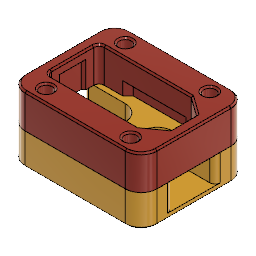
Wiring Box v13 (Autodesk Fusion 360 archive; units mm, degrees)
design "XT90 Mount"
Autodesk Fusion 360 part; units mm, degrees
sketch "Sketch1" plane through (0, 0, 0) normal (0, 0, 1) x (1, 0, 0) in component "Top"
  line L0 (12.5, -10) -> (-12.5, -10)
  line L1 (-12.5, -10) -> (-12.5, 10)
  line L2 (-12.5, 10) -> (12.5, 10)
  line L3 (12.5, 10) -> (12.5, -10)
  line L4 (12.5, -10) -> (-12.5, 10) construction
  line L5 (-12.5, -10) -> (12.5, 10) construction
  line L6 (-10.5, 5) -> (-10.5, -5)
  line L7 (-10.5, -5) -> (7, -5)
  line L8 (7, -5) -> (10.5, -2.5)
  line L9 (10.5, -2.5) -> (10.5, 2.5)
  line L10 (10.5, 2.5) -> (7, 5)
  line L11 (7, 5) -> (-10.5, 5)
  line L12 (0, 0) -> (-22, 0) construction
  line L13 (0, 0) -> (0, 9) construction
  dimension "d1" = 25
  dimension "d2" = 20
  dimension "d3" = 10
  dimension "d4" = 21
  dimension "d5" = 2.5
  dimension "d6" = 3.5
  constraint horizontal L0
  constraint perpendicular L0 L1
  constraint parallel L0 L2
  constraint parallel L1 L3
  constraint coincident L4 L12.start
  constraint coincident L5 L12.start
  constraint coincident L12.start L13.start
  constraint vertical L6
  constraint horizontal L11
  constraint horizontal L7
  constraint vertical L9
  constraint horizontal L12
  constraint symmetric L7 L11 L12
  constraint perpendicular L12 L13
  constraint symmetric L8 L10 L12
  measures "d1" distance of L1.end L2.end
  measures "d2" distance of L0.end L1.end
  measures "d3" distance of L6.start L6.end
  measures "d4" distance of L6 L9
  measures "d5" vertical distance of L9.end L10.end
  measures "d6" horizontal distance of L9.end L10.end
extrude "Extrude1" add sketch "Sketch1" against normal blind 1.5 makes body 1 in component "Top"
fillet "Fillet1" radius 1 2 edges at (-10.5, 5, -0.75) (-10.5, -5, -0.75) on bodies 1 in component "Top"
sketch "Sketch2" plane through (0, 0, -1.5) normal (0, 0, -1) x (1, 0, 0) in component "Top"
  line L0 (7, -5) -> (-9.5, -5)
  arc A0 (-10.5, -4) -> (-9.5, -5) centre (-9.5, -4) ccw
  line L1 (-10.5, -4) -> (-10.5, 4)
  arc A1 (-9.5, 5) -> (-10.5, 4) centre (-9.5, 4) ccw
  line L2 (-9.5, 5) -> (7, 5)
  line L3 (7, 5) -> (10.5, 2.5)
  line L4 (10.5, 2.5) -> (10.5, -2.5)
  line L5 (10.5, -2.5) -> (7, -5)
  line L6 (-12.5, -10) -> (12.5, -10)
  line L7 (12.5, -10) -> (12.5, 10)
  line L8 (12.5, 10) -> (-12.5, 10)
  line L9 (-12.5, 10) -> (-12.5, -10)
  line L10 (10.5, 2.5) -> (11, 2.1429)
  line L11 (11, 2.1429) -> (11, -2.1429)
  line L12 (11, -2.1429) -> (10.5, -2.5)
  line L13 (0, 0) -> (0, 13.3423) construction
  line L14 (-10.5, 2.5) -> (-11, 2.1429)
  line L15 (-11, 2.1429) -> (-11, -2.1429)
  line L16 (-11, -2.1429) -> (-10.5, -2.5)
  dimension "d11" = 0.5
  constraint coincident L3.end L4.start
  constraint parallel L3 L10
  constraint coincident L4.end L5.start
  constraint coincident L13.start origin
  constraint vertical L13
  constraint parallel L5 L12
  constraint vertical L11
  constraint symmetric L3.end L13 L14.start
  constraint symmetric L10.end L13 L14.end
  constraint symmetric L11.end L13 L15.end
  constraint symmetric L4.end L13 L16.end
  measures "d11" distance of L4 L11
extrude "Extrude2" add sketch "Sketch2" along normal blind 2.5 bodies 1 in component "Top"
sketch "Sketch3" plane through (0, 0, -4) normal (0, 0, -1) x (1, 0, 0) in component "Top"
  line L0 (-11, 2.1429) -> (-10.5, 2.5)
  line L1 (-10.5, 2.5) -> (-10.5, 4)
  arc A0 (-9.5, 5) -> (-10.5, 4) centre (-9.5, 4) ccw
  line L2 (-9.5, 5) -> (7, 5)
  line L3 (7, 5) -> (11, 2.1429)
  line L4 (11, 2.1429) -> (11, -2.1429)
  line L5 (11, -2.1429) -> (7, -5)
  line L6 (7, -5) -> (-9.5, -5)
  arc A1 (-10.5, -4) -> (-9.5, -5) centre (-9.5, -4) ccw
  line L7 (-10.5, -4) -> (-10.5, -2.5)
  line L8 (-10.5, -2.5) -> (-11, -2.1429)
  line L9 (-11, -2.1429) -> (-11, 2.1429)
  line L10 (-12.5, 10) -> (-12.5, -10)
  line L11 (-12.5, -10) -> (12.5, -10)
  line L12 (12.5, -10) -> (12.5, 10)
  line L13 (12.5, 10) -> (-12.5, 10)
  line L14 (0, 0) -> (13.5, 0) construction
  line L15 (6, 5) -> (5, 6)
  line L16 (5, 6) -> (-5, 6)
  line L17 (-5, 6) -> (-6, 5)
  line L18 (0, 0) -> (0, 13.6584) construction
  line L19 (6, -5) -> (5, -6)
  line L20 (5, -6) -> (-5, -6)
  line L21 (-5, -6) -> (-6, -5)
  dimension "d17" = 1
  dimension "d18" = 135
  dimension "d19" = 10
  constraint coincident L14.start L18.start
  constraint perpendicular L12 L14
  constraint coincident L2 L15.start
  constraint parallel L2 L16
  constraint coincident L2 L17.end
  constraint perpendicular L13 L18
  constraint symmetric L15 L17 L18
  constraint symmetric L14 L15.start L19.start
  constraint symmetric L14 L15.end L19.end
  constraint symmetric L14 L16.end L20.end
  constraint symmetric L14 L17.end L21.end
  measures "d17" distance of L2 L16
  measures "d18" angle of L15 L16
  measures "d19" distance of L15.end L16.end
extrude "Extrude3" add sketch "Sketch3" along normal blind 2.5 bodies 1 in component "Top"
sketch "Sketch4" plane through (0, 0, 0) normal (0, 0, 1) x (-1, 0, 0) in component "Top"
  line L0 (9.5, -5) -> (-7, -5)
  line L1 (-7, -5) -> (-10.5, -2.5)
  line L2 (-10.5, -2.5) -> (-10.5, 2.5)
  line L3 (-10.5, 2.5) -> (-7, 5)
  line L4 (-7, 5) -> (9.5, 5)
  arc A0 (10.5, 4) -> (9.5, 5) centre (9.5, 4) ccw
  line L5 (10.5, 4) -> (10.5, -4)
  arc A1 (9.5, -5) -> (10.5, -4) centre (9.5, -4) ccw
  line L6 (-12.5, -10) -> (12.5, -10)
  line L7 (12.5, -10) -> (12.5, 10)
  line L8 (12.5, 10) -> (-12.5, 10)
  line L9 (-12.5, 10) -> (-12.5, -10)
  circle A2 centre (8, -7.5) radius 1.15
  line L10 (0, 0) -> (0, -18) construction
  circle A3 centre (-8, -7.5) radius 1.15
  line L11 (0, 0) -> (-17, 0) construction
  circle A4 centre (-8, 7.5) radius 1.15
  circle A5 centre (8, 7.5) radius 1.15
  dimension "d20" = 2.3
  dimension "d21" = 16
  dimension "d22" = 15
  constraint coincident L10.start L11.start
  constraint vertical L10
  constraint symmetric A2 L10 A3
  constraint perpendicular L10 L11
  constraint symmetric A2 L11 A5
  constraint symmetric A3 L11 A4
  measures "d20" diameter of A2
  measures "d21" distance of A2.centre A3.centre
  measures "d22" distance of A3.centre A4.centre
extrude "Extrude4" cut sketch "Sketch4" against normal up to surface (6.5 mm away) contours A2 | A3 | A4 | A5 bodies 1 in component "Top"
fillet "Fillet2" radius 3 4 edges at (-12.5, -10, -3.25) (12.5, -10, -3.25) (12.5, 10, -3.25) (-12.5, 10, -3.25) on bodies 1 in component "Top"
chamfer "Chamfer1" distance 0.3 angle 45 1 faces at (10.6143, -5.4059, 0) on bodies 1 in component "Top"
sketch "Sketch1 (2)" plane through (0, 0, 0) normal (0, 0, 1) x (1, 0, 0) in component "Bottom"
  arc A0 (12.5, 7) -> (9.5, 10) centre (9.5, 7) ccw
  arc A1 (12.5, 7) -> (9.5, 10) centre (9.5, 7) ccw
  line L0 (-9.5, 10) -> (9.5, 10)
  line L1 (9.5, 10) -> (-9.5, 10)
  arc A2 (-9.5, 10) -> (-12.5, 7) centre (-9.5, 7) ccw
  arc A3 (-9.5, 10) -> (-12.5, 7) centre (-9.5, 7) ccw
  line L2 (-12.5, -7) -> (-12.5, 7)
  line L3 (-12.5, 7) -> (-12.5, -7)
  arc A4 (-12.5, -7) -> (-9.5, -10) centre (-9.5, -7) ccw
  arc A5 (-12.5, -7) -> (-9.5, -10) centre (-9.5, -7) ccw
  line L4 (9.5, -10) -> (-9.5, -10)
  line L5 (-9.5, -10) -> (9.5, -10)
  arc A6 (9.5, -10) -> (12.5, -7) centre (9.5, -7) ccw
  arc A7 (9.5, -10) -> (12.5, -7) centre (9.5, -7) ccw
  line L6 (12.5, 7) -> (12.5, -7)
  line L7 (12.5, -7) -> (12.5, 7)
  circle A8 centre (8, 7.5) radius 1.15
  circle A9 centre (8, 7.5) radius 1.15
  circle A10 centre (8, -7.5) radius 1.15
  circle A11 centre (8, -7.5) radius 1.15
  circle A12 centre (-8, -7.5) radius 1.15
  circle A13 centre (-8, -7.5) radius 1.15
  circle A14 centre (-8, 7.5) radius 1.15
  circle A15 centre (-8, 7.5) radius 1.15
  line L8 (-12.5, -4) -> (12.5, -4)
  line L9 (12.5, 4) -> (-12.5, 4)
  line L10 (-1.5, -4) -> (-1.5, 4)
  line L11 (1.5, -4) -> (1.5, 4)
  line L12 (0, 0) -> (0, -8) construction
  line L13 (0, 0) -> (14, 0) construction
  dimension "d28" = 8
  dimension "d29" = 3
  constraint coincident L2 L8.start
  constraint coincident L6 L8.end
  constraint perpendicular L6 L8
  constraint coincident L7 L9.start
  constraint coincident L3 L9.end
  constraint perpendicular L3 L9
  constraint coincident L8 L10.start
  constraint coincident L9 L10.end
  constraint perpendicular L9 L10
  constraint coincident L8 L11.start
  constraint coincident L9 L11.end
  constraint perpendicular L9 L11
  constraint coincident L12.start L13.start
  constraint perpendicular L9 L12
  constraint perpendicular L12 L13
  constraint symmetric L8 L9 L13
  measures "d28" distance of L8 L9
  measures "d29" distance of L10 L11
extrude "Extrude1'" add sketch "Sketch1 (2)" along normal blind 5 separate body contours A0 A1 L0 L1 A2 A3 L2 L3 L6 L7 L9 | L2 L3 A4 A5 L4 L5 A6 A7 L6 L7 L8 | L8 L9 L10 L11 makes body 2 in component "Bottom"
fillet "Fillet1'" radius 3 4 edges at (-1.5, -4, 2.5) (-1.5, 4, 2.5) (1.5, -4, 2.5) (1.5, 4, 2.5) on bodies 2 in component "Bottom"
fillet "Fillet2'" radius 1 4 edges at (-12.5, -4, 2.5) (-12.5, 4, 2.5) (12.5, -4, 2.5) (12.5, 4, 2.5) on bodies 2 in component "Bottom"
sketch "Sketch2 (2)" plane through (0, 0, 0) normal (0, 0, -1) x (1, 0, 0) in component "Bottom"
  arc A0 (12.5, -5) -> (11.5, -4) centre (11.5, -5) ccw
  line L0 (11.5, -4) -> (4.5, -4)
  arc A1 (1.5, -1) -> (4.5, -4) centre (4.5, -1) ccw
  line L1 (1.5, -1) -> (1.5, 1)
  arc A2 (4.5, 4) -> (1.5, 1) centre (4.5, 1) ccw
  line L2 (4.5, 4) -> (11.5, 4)
  arc A3 (11.5, 4) -> (12.5, 5) centre (11.5, 5) ccw
  line L3 (12.5, 5) -> (12.5, 7)
  arc A4 (12.5, 7) -> (9.5, 10) centre (9.5, 7) ccw
  line L4 (9.5, 10) -> (-9.5, 10)
  arc A5 (-9.5, 10) -> (-12.5, 7) centre (-9.5, 7) ccw
  line L5 (-12.5, 7) -> (-12.5, 5)
  arc A6 (-12.5, 5) -> (-11.5, 4) centre (-11.5, 5) ccw
  line L6 (-11.5, 4) -> (-4.5, 4)
  arc A7 (-1.5, 1) -> (-4.5, 4) centre (-4.5, 1) ccw
  line L7 (-1.5, 1) -> (-1.5, -1)
  arc A8 (-4.5, -4) -> (-1.5, -1) centre (-4.5, -1) ccw
  line L8 (-4.5, -4) -> (-11.5, -4)
  arc A9 (-11.5, -4) -> (-12.5, -5) centre (-11.5, -5) ccw
  line L9 (-12.5, -5) -> (-12.5, -7)
  arc A10 (-12.5, -7) -> (-9.5, -10) centre (-9.5, -7) ccw
  line L10 (-9.5, -10) -> (9.5, -10)
  arc A11 (9.5, -10) -> (12.5, -7) centre (9.5, -7) ccw
  line L11 (12.5, -7) -> (12.5, -5)
  circle A12 centre (8, 7.5) radius 1.15
  circle A13 centre (8, -7.5) radius 1.15
  circle A14 centre (-8, 7.5) radius 1.15
  circle A15 centre (-8, -7.5) radius 1.15
  line L12 (-12.5, -5) -> (-12.5, 5)
  line L13 (12.5, -5) -> (12.5, 5)
  constraint coincident A9.end L9.start
  constraint coincident L5.end A6.start
  constraint coincident A0.start L11.end
  constraint coincident A3.end L3.start
extrude "Extrude2'" add sketch "Sketch2 (2)" along normal blind 1 bodies 2 in component "Bottom"
chamfer "Chamfer1'" distance 0.3 angle 45 1 faces at (-2.3857, 2.2393, -1) on bodies 2 in component "Bottom"
component "Top" placed x (1, 0, 0) y (0, 1, 0) z (0, 0, 1) at (0, 0, 0)
component "Bottom" placed x (1, 0, 0) y (0, 1, 0) z (0, 0, 1) at (0, 0, -11.5)

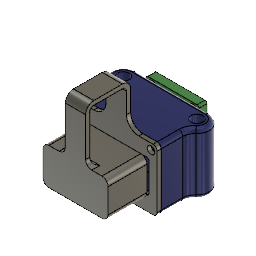
design "XT60 Mount"
Autodesk Fusion 360 part; units mm, degrees
sketch "Sketch1" plane through (0, 0, 0) normal (0, 1, 0) x (1, 0, 0) in component "Outer"
  line L0 (10, 7.5) -> (-10, 7.5)
  line L1 (-10, 7.5) -> (-10, -7.5)
  line L2 (-10, -7.5) -> (10, -7.5)
  line L3 (10, -7.5) -> (10, 7.5)
  line L4 (10, 7.5) -> (-10, -7.5) construction
  line L5 (-10, 7.5) -> (10, -7.5) construction
  line L6 (8, 4) -> (-8, 4)
  line L7 (-8, 4) -> (-8, -4)
  line L8 (-8, -4) -> (8, -4)
  line L9 (8, -4) -> (8, 4)
  line L10 (8, 4) -> (-8, -4) construction
  line L11 (-8, 4) -> (8, -4) construction
  dimension "d1" = 20
  dimension "d2" = 15
  dimension "d3" = 16
  dimension "d4" = 8
  constraint horizontal L0
  constraint perpendicular L0 L1
  constraint parallel L0 L2
  constraint parallel L1 L3
  constraint coincident L4 origin
  constraint coincident L5 origin
  constraint horizontal L6
  constraint perpendicular L6 L7
  constraint parallel L6 L8
  constraint parallel L7 L9
  constraint coincident L10 origin
  constraint coincident L11 origin
  measures "d1" distance of L1.end L2.end
  measures "d2" distance of L0.end L1.end
  measures "d3" distance of L7.end L8.end
  measures "d4" distance of L6.end L7.end
extrude "Extrude1" add sketch "Sketch1" along normal blind 4 makes body 1 in component "Outer"
fillet "Fillet1" radius 0.5 2 edges at (8, 2, -4) (8, 2, 4) on bodies 1 in component "Outer"
fillet "Fillet1" radius 2.5 2 edges at (-8, 2, 4) (-8, 2, -4) on bodies 1 in component "Outer"
sketch "Sketch2" plane through (0, 4, 0) normal (0, 1, 0) x (-1, 0, 0) in component "Outer"
  line L0 (-8, -3.5) -> (-8, 3.5)
  arc A0 (-7.5, 4) -> (-8, 3.5) centre (-7.5, 3.5) ccw
  line L1 (-7.5, 4) -> (5.5, 4)
  arc A1 (8, 1.5) -> (5.5, 4) centre (5.5, 1.5) ccw
  line L2 (8, 1.5) -> (8, -1.5)
  arc A2 (5.5, -4) -> (8, -1.5) centre (5.5, -1.5) ccw
  line L3 (5.5, -4) -> (-7.5, -4)
  arc A3 (-8, -3.5) -> (-7.5, -4) centre (-7.5, -3.5) ccw
  line L4 (-10, 7.5) -> (-10, -7.5)
  line L5 (-10, -7.5) -> (10, -7.5)
  line L6 (10, -7.5) -> (10, 7.5)
  line L7 (10, 7.5) -> (-10, 7.5)
  line L8 (8.25, -4.625) -> (-8.25, -4.625)
  line L9 (-8.25, -4.625) -> (-8.25, 4.625)
  line L10 (-8.25, 4.625) -> (8.25, 4.625)
  line L11 (8.25, 4.625) -> (8.25, -4.625)
  line L12 (8.25, -4.625) -> (-8.25, 4.625) construction
  line L13 (-8.25, -4.625) -> (8.25, 4.625) construction
  dimension "d11" = 16.5
  dimension "d12" = 9.25
  constraint horizontal L8
  constraint perpendicular L8 L9
  constraint parallel L8 L10
  constraint parallel L9 L11
  constraint coincident L12 origin
  constraint coincident L13 origin
  measures "d11" distance of L9.end L10.end
  measures "d12" distance of L8.end L9.end
extrude "Extrude2" add sketch "Sketch2" along normal blind 8.75 contours L4 L5 L6 L7 bodies 1 in component "Outer"
fillet "Fillet2" radius 1.5 4 edges at (-8.25, 8.375, -4.625) (-8.25, 8.375, 4.625) (8.25, 8.375, 4.625) (8.25, 8.375, -4.625) on bodies 1 in component "Outer"
sketch "Sketch3" plane through (0, 0, 7.5) normal (0, 0, 1) x (-1, 0, 0) in component "Outer"
  line L0 (10, 0) -> (-10, 0)
  line L1 (-10, 0) -> (-10, -12.75)
  line L2 (-10, -12.75) -> (10, -12.75)
  line L3 (10, -12.75) -> (10, 0)
  circle A0 centre (9, -9.75) radius 1.425
  circle A1 centre (-9, -9.75) radius 1.425
  line L4 (0, 0) -> (0, -18.4938) construction
  circle A2 centre (9, -9.75) radius 3
  circle A3 centre (-9, -9.75) radius 3
  dimension "d17" = 9.75
  dimension "d18" = 9
  dimension "d19" = 2.85
  dimension "d20" = 6
  constraint coincident L4.start origin
  constraint perpendicular L0 L4
  constraint concentric A0 A2
  constraint symmetric A0 A1 L4
  constraint symmetric L4 A2 A3
  measures "d17" distance of L0 A0.centre
  measures "d18" distance of A0.centre L4
  measures "d19" diameter of A0
  measures "d20" diameter of A2
extrude "Extrude3" add sketch "Sketch3" against normal up to surface (15 mm away) contours L3 A0 A2 | L1 A1 A3 picked at (10.7902, -8.0482) picked at (-10.8276, -8.0902) bodies 1 in component "Outer"
extrude "Extrude4" cut sketch "Sketch3" against normal up to surface (15 mm away) contours L3 A0 | L2 L3 A2 | L1 A1 | L1 L2 A3 picked at (9.1917, -9.75) picked at (-9.368, -9.2983) bodies 1 in component "Outer"
fillet "Fillet3" radius 3 2 edges at (10, 6.9216, 0) (-10, 6.9216, 0) on bodies 1 in component "Outer"
sketch "Sketch4" plane through (0, 12.75, 0) normal (0, 1, 0) x (-1, 0, 0) in component "Outer"
  line L0 (-9, 7.5) -> (-9, -7.5)
  line L1 (-9, -7.5) -> (9, -7.5)
  line L2 (9, -7.5) -> (9, 7.5)
  line L3 (9, 7.5) -> (-9, 7.5)
  line L4 (-6.75, 4.625) -> (6.75, 4.625)
  arc A0 (8.25, 3.125) -> (6.75, 4.625) centre (6.75, 3.125) ccw
  line L5 (8.25, 3.125) -> (8.25, -3.125)
  arc A1 (6.75, -4.625) -> (8.25, -3.125) centre (6.75, -3.125) ccw
  line L6 (6.75, -4.625) -> (-6.75, -4.625)
  arc A2 (-8.25, -3.125) -> (-6.75, -4.625) centre (-6.75, -3.125) ccw
  line L7 (-8.25, -3.125) -> (-8.25, 3.125)
  arc A3 (-6.75, 4.625) -> (-8.25, 3.125) centre (-6.75, 3.125) ccw
  line L8 (0, 0) -> (0, 8) construction
  line L9 (0, 0) -> (15, 0) construction
  circle A4 centre (-5, 6) radius 0.925
  circle A5 centre (5, 6) radius 0.925
  circle A6 centre (5, -6) radius 0.925
  circle A7 centre (-5, -6) radius 0.925
  dimension "d27" = 1.85
  dimension "d28" = 1.5
  dimension "d29" = 5
  constraint coincident L8.start L9.start
  constraint vertical L8
  constraint perpendicular L8 L9
  constraint symmetric L8 A4 A5
  constraint symmetric L9 A4 A7
  constraint symmetric L9 A5 A6
  measures "d27" diameter of A4
  measures "d28" distance of L3 A4.centre
  measures "d29" distance of L8 A4.centre
extrude "Extrude5" cut sketch "Sketch4" against normal blind 5 contours A4 | A5 | A6 | A7 bodies 1 in component "Outer"
sketch "Sketch5" plane through (0, 0, 0) normal (0, -1, 0) x (1, 0, 0) in component "Outer"
  arc A0 (7.5, -4) -> (8, -3.5) centre (7.5, -3.5) ccw
  line L0 (7.5, -4) -> (-5.5, -4)
  arc A1 (-8, -1.5) -> (-5.5, -4) centre (-5.5, -1.5) ccw
  line L1 (-8, -1.5) -> (-8, 1.5)
  arc A2 (-5.5, 4) -> (-8, 1.5) centre (-5.5, 1.5) ccw
  line L2 (-5.5, 4) -> (7.5, 4)
  arc A3 (8, 3.5) -> (7.5, 4) centre (7.5, 3.5) ccw
  line L3 (8, 3.5) -> (8, -3.5)
  line L4 (10, -7.5) -> (10, 7.5)
  line L5 (10, 7.5) -> (-10, 7.5)
  line L6 (-10, 7.5) -> (-10, -7.5)
  line L7 (-10, -7.5) -> (10, -7.5)
  circle A4 centre (8.5, 6) radius 0.925
  line L8 (0, 0) -> (0, 11.5757) construction
  circle A5 centre (-8.5, 6) radius 0.925
  dimension "d37" = 1.85
  dimension "d38" = 1.5
  dimension "d39" = 8.5
  constraint coincident L8.start origin
  constraint perpendicular L5 L8
  constraint symmetric A4 L8 A5
  measures "d37" diameter of A4
  measures "d38" distance of L5 A4.centre
  measures "d39" distance of A4.centre L8
extrude "Extrude6" cut sketch "Sketch5" against normal blind 6 contours A4 | A5 bodies 1 in component "Outer"
fillet "Fillet4" radius 1 14 edges at (-10, 2.6389, 7.5) (-10.2614, 6.5026, 7.5) (-11.8025, 10.8205, 7.5) (0, 12.75, 7.5) (11.8025, 10.8205, 7.5) (10.2614, 6.5026, 7.5) (10, 2.6389, 7.5) (10, 2.6389, -7.5) (10.2614, 6.5026, -7.5) (11.8025, 10.8205, -7.5) (0, 12.75, -7.5) (-11.8025, 10.8205, -7.5) (-10.2614, 6.5026, -7.5) (-10, 2.6389, -7.5) on bodies 1 in component "Outer"
sketch "Sketch1 (2)" plane through (0, 0, 0) normal (0, 1, 0) x (1, 0, 0) in component "Inner"
  spline S0 degree 3 poles (-4.2218, -6.5) (-4.264, -6.5657) (-4.3178, -6.6288) (-4.4519, -6.7533) (-4.5521, -6.8178) (-4.7704, -6.9037) (-4.8885, -6.925) (-5, -6.925) (-5.1115, -6.925) (-5.2296, -6.9037) (-5.4479, -6.8178) (-5.5481, -6.7533) (-5.6822, -6.6288) (-5.736, -6.5657) (-5.7782, -6.5) knots 0.89406 0.89406 0.89406 0.89406 0.915914 0.915914 0.949353 0.949353 0.982793 0.982793 0.982793 1.016232 1.016232 1.049672 1.049672 1.071526 1.071526 1.071526 1.071526
  arc A0 (-4.2218, -6.5) -> (-5.7782, -6.5) centre (-5, -6) ccw
  circle A1 centre (-5, -6) radius 0.925
  spline S1 degree 3 poles (5.7782, -6.5) (5.736, -6.5657) (5.6822, -6.6288) (5.5481, -6.7533) (5.4479, -6.8178) (5.2296, -6.9037) (5.1115, -6.925) (5, -6.925) (4.8885, -6.925) (4.7704, -6.9037) (4.5521, -6.8178) (4.4519, -6.7533) (4.3178, -6.6288) (4.264, -6.5657) (4.2218, -6.5) knots 0.89406 0.89406 0.89406 0.89406 0.915914 0.915914 0.949353 0.949353 0.982793 0.982793 0.982793 1.016232 1.016232 1.049672 1.049672 1.071526 1.071526 1.071526 1.071526
  arc A2 (5.7782, -6.5) -> (4.2218, -6.5) centre (5, -6) ccw
  circle A3 centre (5, -6) radius 0.925
  line L0 (6.5, -7.5) -> (6.5, -3.3)
  line L1 (6.5, -3.3) -> (-6.5, -3.3)
  line L2 (-6.5, -3.3) -> (-6.5, -7.5)
  line L3 (-6.5, -7.5) -> (6.5, -7.5)
  line L4 (6.5, -4.5) -> (-6.5, -4.5)
  line L5 (0, 0) -> (0, -11.2972) construction
  circle A4 centre (5, -6) radius 1.15
  circle A5 centre (-5, -6) radius 1.15
  dimension "d42" = 1.5
  dimension "d43" = 1.2
  dimension "d45" = 1.5
  dimension "d46" = 13
  dimension "d47" = 2.3
  constraint vertical L0
  constraint perpendicular L0 L1
  constraint perpendicular L1 L2
  constraint coincident L0 L4.start
  constraint coincident L2 L4.end
  constraint perpendicular L2 L4
  constraint horizontal L3
  constraint coincident L5.start origin
  constraint perpendicular L1 L5
  constraint symmetric L0 L2 L5
  constraint concentric A2 A4
  constraint concentric A0 A5
  constraint equal A4 A5
  measures "d42" distance of A0.centre L4
  measures "d43" distance of L1 L4
  measures "d45" distance of A0.centre L3
  measures "d46" distance of L0.start L2.end
  measures "d47" diameter of A4
extrude "Extrude1'" add sketch "Sketch1 (2)" along normal blind 2 separate body contours L0 L2 L3 L4 | L0 L1 L2 L4 makes body 2 in component "Inner"
extrude "Extrude2'" add sketch "Sketch1 (2)" against normal up to surface (4.75 mm away) contours L0 L1 L2 L4 bodies 2 in component "Inner"
fillet "Fillet1'" radius 0.5 6 edges at (6.5, -1.375, 3.3) (6.5, 1, 7.5) (-6.5, 1, 7.5) (-6.5, -1.375, 3.3) (6.5, -2.375, 4.5) (-6.5, -2.375, 4.5) on bodies 2 in component "Inner"
fillet "Fillet2'" radius 0.2 3 edges at (-6.3536, 0, 4.3536) (0, 0, 4.5) (6.3536, 0, 4.3536) on bodies 2 in component "Inner"
sketch "Sketch1 (3)" plane through (0, 0, 0) normal (0, -1, 0) x (1, 0, 0) in component "Cover"
  circle A0 centre (8.5, 6) radius 0.925
  circle A1 centre (-8.5, 6) radius 0.925
  arc A2 (7.5, -4) -> (8, -3.5) centre (7.5, -3.5) ccw
  line L0 (7.5, -4) -> (-5.5, -4)
  arc A3 (-8, -1.5) -> (-5.5, -4) centre (-5.5, -1.5) ccw
  line L1 (-8, -1.5) -> (-8, 1.5)
  arc A4 (-5.5, 4) -> (-8, 1.5) centre (-5.5, 1.5) ccw
  line L2 (-5.5, 4) -> (7.5, 4)
  arc A5 (8, 3.5) -> (7.5, 4) centre (7.5, 3.5) ccw
  line L3 (8, 3.5) -> (8, -3.5)
  arc A6 (9, -7.5) -> (10, -6.5) centre (9, -6.5) ccw
  line L4 (10, -6.5) -> (10, 6.5)
  arc A7 (10, 6.5) -> (9, 7.5) centre (9, 6.5) ccw
  line L5 (9, 7.5) -> (-9, 7.5)
  arc A8 (-9, 7.5) -> (-10, 6.5) centre (-9, 6.5) ccw
  line L6 (-10, 6.5) -> (-10, -6.5)
  arc A9 (-10, -6.5) -> (-9, -7.5) centre (-9, -6.5) ccw
  line L7 (-9, -7.5) -> (9, -7.5)
  line L8 (-2.5, 7.5) -> (-2.5, 17.5)
  line L9 (-2.5, 17.5) -> (2.5, 17.5)
  line L10 (2.5, 17.5) -> (2.5, 7.5)
  line L11 (0, 0) -> (0, 17) construction
  dimension "d61" = 5
  dimension "d62" = 10
  constraint coincident L5 L8.start
  constraint perpendicular L5 L8
  constraint perpendicular L8 L9
  constraint coincident L5 L10.end
  constraint perpendicular L5 L10
  constraint coincident L11.start origin
  constraint perpendicular L9 L11
  measures "d61" distance of L8.end L9.end
  measures "d62" distance of L5 L9
extrude "Extrude1''" add sketch "Sketch1 (3)" along normal blind 1 separate body makes body 3 in component "Cover"
sketch "Sketch2 (2)" plane through (0, -1, 0) normal (0, -1, 0) x (1, 0, 0) in component "Cover"
  line L0 (2.5, 7.5) -> (2.5, 17.5)
  line L1 (2.5, 17.5) -> (-2.5, 17.5)
  line L2 (-2.5, 17.5) -> (-2.5, 7.5)
  line L3 (-2.5, 7.5) -> (-9, 7.5)
  line L4 (-2.5, 16.5) -> (2.5, 16.5)
  arc A0 (-5.5, 4) -> (-8, 1.5) centre (-5.5, 1.5) ccw
  line L5 (-5.5, 4) -> (7.5, 4)
  arc A1 (8, 3.5) -> (7.5, 4) centre (7.5, 3.5) ccw
  line L6 (8, 3.5) -> (8, -3.5)
  arc A2 (7.5, -4) -> (8, -3.5) centre (7.5, -3.5) ccw
  line L7 (7.5, -4) -> (-5.5, -4)
  arc A3 (-8, -1.5) -> (-5.5, -4) centre (-5.5, -1.5) ccw
  line L8 (-8, -1.5) -> (-8, 1.5)
  circle A4 centre (-8.5, 6) radius 0.925
  circle A5 centre (8.5, 6) radius 0.925
  arc A6 (-9, 7.5) -> (-10, 6.5) centre (-9, 6.5) ccw
  line L9 (-10, 6.5) -> (-10, -6.5)
  arc A7 (-10, -6.5) -> (-9, -7.5) centre (-9, -6.5) ccw
  line L10 (-9, -7.5) -> (9, -7.5)
  arc A8 (9, -7.5) -> (10, -6.5) centre (9, -6.5) ccw
  line L11 (10, -6.5) -> (10, 6.5)
  arc A9 (10, 6.5) -> (9, 7.5) centre (9, 6.5) ccw
  line L12 (9, 7.5) -> (2.5, 7.5)
  dimension "d71" = 1
  constraint coincident L2 L4.start
  constraint coincident L0 L4.end
  constraint perpendicular L0 L4
  measures "d71" distance of L1 L4
extrude "Extrude2''" add sketch "Sketch2 (2)" along normal blind 9 contours L0 L1 L2 L4 bodies 3 in component "Cover"
sketch "Sketch3 (2)" plane through (0, -10, 0) normal (0, -1, 0) x (1, 0, 0) in component "Cover"
  line L0 (-2.5, 16.5) -> (2.5, 16.5)
  line L1 (2.5, 16.5) -> (2.5, 17.5)
  line L2 (2.5, 17.5) -> (-2.5, 17.5)
  line L3 (-2.5, 17.5) -> (-2.5, 16.5)
  line L4 (7, 3.5) -> (-7, 3.5)
  line L5 (-7, 3.5) -> (-7, -3.5)
  line L6 (-7, -3.5) -> (7, -3.5)
  line L7 (7, -3.5) -> (7, 3.5)
  line L8 (7, 3.5) -> (-7, -3.5) construction
  line L9 (-7, 3.5) -> (7, -3.5) construction
  line L10 (2.5, 16.5) -> (2.5, 4.5)
  line L11 (8, 4.5) -> (8, -4.5)
  line L12 (8, -4.5) -> (-8, -4.5)
  line L13 (-8, -4.5) -> (-8, 4.5)
  line L14 (-2.5, 4.5) -> (-2.5, 16.5)
  line L15 (-8, 4.5) -> (8, 4.5)
  dimension "d74" = 14
  dimension "d75" = 7
  dimension "d77" = 1
  dimension "d78" = 1
  dimension "d79" = 1
  dimension "d84" = 1
  constraint horizontal L4
  constraint perpendicular L4 L5
  constraint parallel L4 L6
  constraint parallel L5 L7
  constraint coincident L8 origin
  constraint coincident L9 origin
  constraint coincident L0.end L1.start
  constraint perpendicular L0 L10
  constraint perpendicular L0 L11
  constraint perpendicular L11 L12
  constraint perpendicular L0 L13
  constraint coincident L0.start L3.end
  constraint vertical L14
  constraint coincident L10.end L15
  constraint coincident L14.start L15
  measures "d74" distance of L5.end L6.end
  measures "d75" distance of L4.end L5.end
  measures "d77" distance of L7 L11
  measures "d78" distance of L6 L12
  measures "d79" distance of L5 L13
  measures "d84" distance of L4 L15
extrude "Extrude3'" add sketch "Sketch3 (2)" along normal blind 1 contours L0 L1 L2 L3 | L0 L10 L14 L15 | L11 L12 L13 L15 | L4 L5 L6 L7 bodies 3 in component "Cover"
extrude "Extrude4'" add sketch "Sketch3 (2)" against normal up to surface (8.5 mm away) contours L11 L12 L13 L15 bodies 3 in component "Cover"
fillet "Fillet2''" radius 3 2 edges at (2.5, -0.5, 7.5) (-2.5, -0.5, 7.5) on bodies 3 in component "Cover"
fillet "Fillet3'" radius 1 3 edges at (0, -1, 16.5) (0, -10, 16.5) (0, -10, 4.5) on bodies 3 in component "Cover"
fillet "Fillet3'" radius 2 2 edges at (0, 0, 17.5) (0, -11, 17.5) on bodies 3 in component "Cover"
fillet "Fillet4'" radius 0.5 4 edges at (7, -5.75, 3.5) (7, -5.75, -3.5) (-7, -5.75, -3.5) (-7, -5.75, 3.5) on bodies 3 in component "Cover"
fillet "Fillet4'" radius 1.5 4 edges at (-8, -6.25, 4.5) (-8, -6.25, -4.5) (8, -6.25, -4.5) (8, -6.25, 4.5) on bodies 3 in component "Cover"
fillet "Fillet5" radius 1.5 2 edges at (-2.5, -10, 4.5) (2.5, -10, 4.5) on bodies 3 in component "Cover"
fillet "Fillet6" radius 0.5 8 edges at (7, -10, 0) (6.8536, -10, -3.3536) (0, -10, -3.5) (-6.8536, -10, -3.3536) (-7, -10, 0) (-6.8536, -10, 3.3536) (0, -10, 3.5) (6.8536, -10, 3.3536) on bodies 3 in component "Cover"
component "Outer" placed x (1, 0, 0) y (0, 1, 0) z (0, 0, 1) at (0, 0, 0)
component "Inner" placed x (1, 0, 0) y (0, 1, 0) z (0, 0, 1) at (0, 12.75, 0)
component "Cover" placed x (1, 0, 0) y (0, 1, 0) z (0, 0, 1) at (0, 0, 0)
equation "d13 = 9.75 mm + 3 mm - 4 mm"
